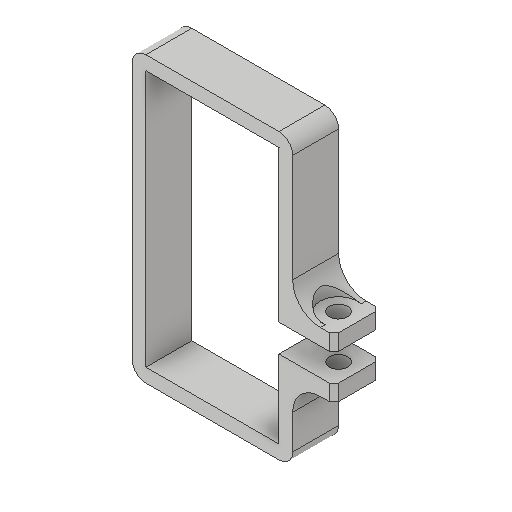
# Autodesk Inventor part: 3DP_PLA_Battery_mount
Saved by Autodesk Inventor 2026.1 (Build 301233000, 233)
## iProperties
Created: 2020-03-29
Part Number: 3DP_PLA_Battery_mount
Material: Generic
Document SubType Name: Modeling
Designer: Andrzej
Density: 1 g/cm^3
Appearance: Default
Author: Andrzej
Autodesk Inventor part; units mm, degrees
note: some values were not read from the file. Chosen so that the rebuilt part matches the saved one: direction of "Hole1".
ref_plane "YZ Plane" through (0, 0, 0) normal (1, 0, 0) x (0, 1, 0)
ref_plane "XZ Plane" through (0, 0, 0) normal (0, 1, 0) x (-1, 0, 0)
ref_plane "XY Plane" through (0, 0, 0) normal (0, 0, 1) x (1, 0, 0)
sketch "Sketch1" plane through (0, 0, 0) normal (0, 0, 1) x (1, 0, 0)
  line L0 (-14.5, 28) -> (14.5, 28)
  line L1 (14.5, 28) -> (14.5, -28)
  line L2 (14.5, -28) -> (-14.5, -28)
  line L3 (-14.5, -28) -> (-14.5, 28)
  line L4 (17.5, 31) -> (-17.5, 31)
  line L5 (-17.5, 31) -> (-17.5, -31)
  line L6 (-17.5, -31) -> (17.5, -31)
  line L7 (14.5, -1.5) -> (26.5, -1.5)
  line L8 (14.5, -14.5) -> (26.5, -14.5)
  line L9 (17.5, -31) -> (17.5, -14.5)
  line L10 (17.5, -1.5) -> (17.5, 31)
  line L11 (26.5, -1.5) -> (26.5, -5)
  line L12 (26.5, -5) -> (14.5, -5)
  line L13 (26.5, -14.5) -> (26.5, -11)
  line L14 (26.5, -11) -> (14.5, -11)
  point P0 (0, 0)
  dimension "d0" = 29
  dimension "d1" = 56
  dimension "d2" = 14.5
  dimension "d3" = 28
  dimension "d4" = 3
  dimension "d5" = 12
  dimension "d6" = 3.5
  dimension "d7" = 3.5
  dimension "d8" = 6
  dimension "d9" = 32.5
  dimension "d10" = 62
  constraints: 30 end point, 6 point on line, 5 parallel, 5 perpendicular, 3 horizontal, 2 vertical, 1 vertical alignment, 2 other
  measures "d0" distance of L1.end L2.end
  measures "d1" distance of L0.end L1.end
  measures "d2" distance from line of L3 point (0, 0)
  measures "d3" distance from line of L0 point (0, 0)
  measures "d4" distance between parallel lines of L0 L4
  measures "d5" distance between parallel lines of L1 L11
  measures "d6" distance between parallel lines of L7 L12
  measures "d7" distance between parallel lines of L14 L8
  measures "d8" distance between parallel lines of L14 L12
  measures "d9" distance between parallel lines of L4 L7
  measures "d10" distance between parallel lines of L6 L4
extrude "Extrusion1" add sketch "Sketch1" along normal blind 10 contours L3 L2 L1 L8 L9 L6 L5 L4 L10 L7 L0 | L7 L11 L12 L1 | L1 L14 L13 L8
sketch "Sketch2" plane through (17.5, -1.5, 0) normal (0, 1, 0) x (1, 0, 0)
  line L0 (0, 0) -> (0, -10) projected
  line L1 (9, -10) -> (0, -10) projected
  line L2 (9, 0) -> (9, -10) projected
  line L3 (9, 0) -> (0, 0) projected
  point P0 (-17.5, 0)
  point P1 (5, -5)
  dimension "d13" = 4
  measures "d13" distance from line of L2 point (5, -5)
hole "Hole1" at (22.5, -1.5, 5) direction (0, -1, 0) diameter 4 depth 13
chamfer "Chamfer1" distance 1 angle 45 4 edges at (26.5, -3.25, 0) (26.5, -3.25, 10) (26.5, -12.75, 10) (26.5, -12.75, 0)
fillet "Fillet1" radius 6 2 edges at (17.5, -14.5, 5) (17.5, -1.5, 5)
sketch "Sketch3" plane through (26.5, -1.5, 9) normal (0, 1, 0) x (1, 0, 0)
  line L0 (-3, -1) -> (-3, 2.2679) projected
  line L1 (-1, -1) -> (-3, -1) projected
  line L2 (0, 0) -> (-1, -1) projected
  line L3 (0, 8) -> (0, 0) projected
  line L4 (-1, 9) -> (0, 8) projected
  line L5 (-1, 9) -> (-3, 9) projected
  line L6 (-3, 5.7321) -> (-3, 9) projected
  arc A0 (-3, 2.2679) -> (-3, 5.7321) centre (-4, 4) ccw projected
  circle A1 centre (-4, 4) radius 4
  point P0 (-26.5, 9)
  dimension "d25" = 8
  constraints: 1 centre point, 1 coincident
  measures "d25" diameter of A1
extrude "Extrusion2" cut sketch "Sketch3" along normal blind 10 contours A1 L6 A0 L0 | L0 A0 L6 A1
sketch "Sketch4" plane through (26.5, -14.5, 1) normal (0, -1, 0) x (1, 0, 0)
  line L0 (-3, -1) -> (-3, 2.2679) projected
  line L1 (-3, -1) -> (-1, -1) projected
  line L2 (0, 0) -> (-1, -1) projected
  line L3 (0, 0) -> (0, 8) projected
  line L4 (-1, 9) -> (0, 8) projected
  line L5 (-3, 9) -> (-1, 9) projected
  line L6 (-3, 5.7321) -> (-3, 9) projected
  arc A0 (-3, 2.2679) -> (-3, 5.7321) centre (-4, 4) ccw projected
  circle A1 centre (-4, 4) radius 4
  point P0 (-26.5, -1)
  dimension "d28" = 8
  constraints: 1 centre point
  measures "d28" diameter of A1
extrude "Extrusion3" cut sketch "Sketch4" along normal blind 10 contours A1 L6 A0 L0 | L0 A0 L6 A1
fillet "Fillet2" radius 3 4 edges at (17.5, 31, 5) (-17.5, 31, 5) (-17.5, -31, 5) (17.5, -31, 5)
equation "\"d2\" = 0.5 * d0"
equation "\"d3\" = 0.5 * d1"
equation "\"d7\" = d6"
body "Solid1"
